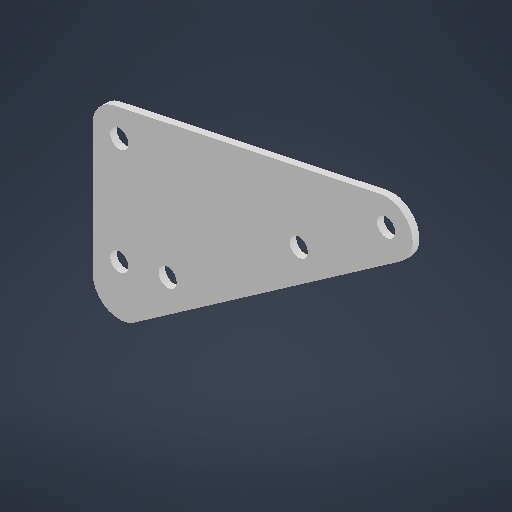
# Autodesk Inventor part: Part4
Saved by Autodesk Inventor 2025.1 (Build 291241000, 241)
## iProperties
Created: 2025-01-15
Part Number: Part4
Material: Generic
Document SubType Name: Modeling
Designer: Jahan
Density: 1 g/cm^3
Appearance: Default
Author: Jahan
Autodesk Inventor part; units mm, degrees
ref_plane "YZ Plane" through (0, 0, 0) normal (1, 0, 0) x (0, 1, 0)
ref_plane "XZ Plane" through (0, 0, 0) normal (0, 1, 0) x (-1, 0, 0)
ref_plane "XY Plane" through (0, 0, 0) normal (0, 0, 1) x (1, 0, 0)
sketch "Sketch1" plane through (0, 0, 0) normal (0, 0, 1) x (1, 0, 0)
  ellipse E0 centre (36.5765, 33.5673) end of major axis (38.7609, 33.5673) minor radius 2.1844
  ellipse E1 centre (15.7624, 19.0472) end of major axis (13.578, 19.0472) minor radius 2.1844
  circle A0 centre (-26.9864, 20.0563) radius 2.1844
  ellipse E2 centre (-15.4587, -2.7897) end of major axis (-17.6431, -2.7897) minor radius 2.1844
  circle A1 centre (-26.9864, -5.3437) radius 2.1844
  line L0 (-33.3154, -10.8959) -> (-33.3364, 20.0563)
  arc A2 (-33.3154, -10.8959) -> (-23.9629, -16.4869) centre (-26.9654, -10.8916) ccw
  line L1 (-28.3066, 26.2675) -> (35.2563, 39.7785)
  line L2 (-23.9629, -16.4869) -> (40.2139, 28.3623)
  arc A3 (40.2139, 28.3623) -> (35.2563, 39.7785) centre (36.5765, 33.5673) ccw
  arc A4 (-28.3066, 26.2675) -> (-33.3364, 20.0563) centre (-26.9864, 20.0563) ccw
  point P0 (0, 0)
  constraints: 6 centre point, 6 end point, 6 point on circle, 2 coincident, 7 other
extrude "Extrusion1" add sketch "Sketch1" along normal blind 1.5875
body "Solid1"
